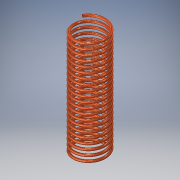
# Autodesk Inventor part: spring
Saved by Autodesk Inventor 2016 (Build 200138000, 138)
## iProperties
Created: 2015-05-24
Part Number: spring
Material: Generic
Document SubType Name: Modeling
Designer: Admin
Density: 1 g/cm^3
Appearance: Default
Author: Admin
Autodesk Inventor part; units mm, degrees
ref_plane "YZ Plane" through (0, 0, 0) normal (1, 0, 0) x (0, 1, 0)
ref_plane "XZ Plane" through (0, 0, 0) normal (0, 1, 0) x (-1, 0, 0)
ref_plane "XY Plane" through (0, 0, 0) normal (0, 0, 1) x (1, 0, 0)
sketch "Sketch3" plane through (0, 0, 0) normal (1, 0, 0) x (0, 1, 0)
  line L0 (0, 0) -> (53.7972, 0)
  line L1 (0, 0) -> (0, -7.62)
  circle A0 centre (0, -7.62) radius 0.635
  dimension "d10" = 53.7972
  dimension "d11" = 7.62
  dimension "d12" = 1.27
  constraints: 4 end point, 1 centre point, 1 coincident, 1 horizontal, 1 vertical
  measures "d10" distance of L0.start L0.end
  measures "d11" distance of L0.start L1.end
  measures "d12" diameter of A0
coil "Coil2" sketch "Sketch3" operation add axis through (0, 0, 0) along (0, 1, 0) pitch 2.54 turns 21.18 hand right
body "Solid2"
